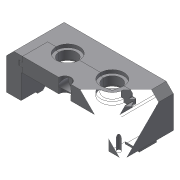
# Autodesk Inventor part: Carriage nozzel Holder
Saved by Autodesk Inventor 2015 (Build 190159000, 159)
## iProperties
Created: 2020-03-28
Part Number: Carriage nozzel Holder
Material: Generic
Document SubType Name: Modeling
Designer: Ghassan Yusuf
Density: 1 g/cm^3
Appearance: Default
Author: Ghassan Yusuf
Autodesk Inventor part; units mm, degrees
ref_plane "YZ Plane" through (0, 0, 0) normal (1, 0, 0) x (0, 1, 0)
ref_plane "XZ Plane" through (0, 0, 0) normal (0, 1, 0) x (-1, 0, 0)
ref_plane "XY Plane" through (0, 0, 0) normal (0, 0, 1) x (1, 0, 0)
sketch "Sketch1" plane through (0, 0, 0) normal (0, 0, 1) x (1, 0, 0)
  line L0 (-40.5, 17.5) -> (40.5, 17.5)
  line L1 (40.5, 17.5) -> (40.5, -17.5)
  line L2 (40.5, -17.5) -> (-40.5, -17.5)
  line L3 (-40.5, -17.5) -> (-40.5, 17.5)
  line L4 (-40.5, 17.5) -> (40.5, -17.5) construction
  line L5 (40.5, 17.5) -> (-40.5, -17.5) construction
  circle A0 centre (-15.5, 0) radius 6.125
  circle A1 centre (15.5, 0) radius 6.125
  point P0 (0, 0)
  dimension "d0" = 81
  dimension "d1" = 35
  dimension "d2" = 12.25
  dimension "d3" = 31
  dimension "d4" = 15.5
  constraints: 12 end point, 2 centre point, 2 midpoint, 2 parallel, 1 equal radius, 1 horizontal, 1 perpendicular
  measures "d0" distance of L1.end L2.end
  measures "d1" distance of L0.end L1.end
  measures "d2" diameter of A0
  measures "d3" distance of A1.centre A0.centre
  measures "d4" distance of point (0, 0) A0.centre
extrude "Extrusion1" add sketch "Sketch1" along normal mid plane 10
sketch "Sketch2" plane through (0, 0, 5) normal (0, 0, 1) x (1, 0, 0)
  circle A0 centre (-15.5, 0) radius 6.125 projected
  circle A1 centre (-15.5, 0) radius 8.125
  circle A2 centre (15.5, 0) radius 6.125 projected
  circle A3 centre (15.5, 0) radius 8.125
  point P0 (0, 0)
  dimension "d7" = 16.25
  dimension "d8" = 16.25
  constraints: 2 centre point, 2 coincident
  measures "d7" diameter of A1
  measures "d8" diameter of A3
extrude "Extrusion2" cut sketch "Sketch2" against normal blind 2.25 contours A0 | A1 | A2 | A3
sketch "Sketch3" plane through (0, 0, -5) normal (0, 0, -1) x (-1, 0, 0)
  circle A0 centre (15.5, 0) radius 8.125 projected
  circle A1 centre (15.5, 0) radius 8.125
  circle A2 centre (-15.5, 0) radius 6.125 projected
  circle A3 centre (-15.5, 0) radius 8.125
  circle A4 centre (-15.5, 0) radius 8.125 projected
  point P0 (0, 0)
  constraints: 2 centre point, 2 coincident, 2 concentric
extrude "Extrusion3" cut sketch "Sketch3" against normal blind 2.25
sketch "Sketch4" plane through (0, 0, 5) normal (0, 0, 1) x (1, 0, 0)
  line L0 (40.5, -17.5) -> (-40.5, -17.5) projected
  line L1 (-40.5, 17.5) -> (-30.5, 17.5)
  line L2 (-30.5, 17.5) -> (-30.5, -17.5)
  line L3 (-30.5, -17.5) -> (-40.5, -17.5)
  line L4 (-40.5, -17.5) -> (-40.5, 17.5)
  line L5 (40.5, 17.5) -> (30.5, 17.5)
  line L6 (30.5, 17.5) -> (30.5, -17.5)
  line L7 (30.5, -17.5) -> (40.5, -17.5)
  line L8 (40.5, -17.5) -> (40.5, 17.5)
  point P0 (0, 0)
  dimension "d13" = 10
  dimension "d14" = 10
  constraints: 16 end point, 4 parallel, 2 horizontal, 2 perpendicular, 2 point on line
  measures "d13" distance of L2.end L3.end
  measures "d14" distance of L7.end L6.end
extrude "Extrusion4" add sketch "Sketch4" along normal blind 17.17
sketch "Sketch5" plane through (0, 0, 22.17) normal (0, 0, 1) x (1, 0, 0)
  line L0 (-40.5, -17.5) -> (-40.5, 17.5) projected
  line L1 (-30.5, -17.5) -> (-30.5, 17.5) projected
  line L2 (-40.5, -6) -> (-30.5, -6)
  line L3 (-30.5, -6) -> (-30.5, 6)
  line L4 (-30.5, 6) -> (-40.5, 6)
  line L5 (-40.5, 6) -> (-40.5, -6)
  line L6 (30.5, 17.5) -> (30.5, -17.5) projected
  line L7 (30.5, -6) -> (40.3218, -6)
  line L8 (40.3218, -6) -> (40.3218, 6)
  line L9 (40.3218, 6) -> (30.5, 6)
  line L10 (30.5, 6) -> (30.5, -6)
  point P0 (0, 0)
  point P1 (-30.5, 0)
  point P2 (30.5, 0)
  dimension "d17" = 12
  constraints: 16 end point, 4 parallel, 3 point on line, 2 collinear, 2 horizontal, 2 horizontal alignment, 2 midpoint, 2 perpendicular
  measures "d17" distance between parallel lines of L4 L2
extrude "Extrusion5" add sketch "Sketch5" along normal blind 1.4
sketch "Sketch6" plane through (0, 0, -5) normal (0, 0, -1) x (-1, 0, 0)
  line L0 (-30.5, 17.5) -> (30.5, 17.5) projected
  circle A0 centre (0, 17.5) radius 4.25
  point P0 (0, 0)
  dimension "d20" = 8.5
  constraints: 1 centre point, 1 midpoint
  measures "d20" diameter of A0
extrude "Extrusion6" cut sketch "Sketch6" against normal blind 12.75
chamfer "Chamfer3" distance 5 angle 45 2 edges at (40.5, 0, -5) (-40.5, 0, -5)
fillet "Fillet4" radius 1 2 edges at (-30.5, 0, 5) (30.5, 0, 5)
sketch "Sketch7" plane through (0, 0, 5) normal (0, 0, 1) x (1, 0, 0)
  line L0 (-29.5, 17.5) -> (29.5, 17.5)
  line L1 (29.5, 17.5) -> (29.5, 0)
  line L2 (29.5, 0) -> (-29.5, 0)
  line L3 (-29.5, 0) -> (-29.5, 17.5)
  line L4 (-29.5, -17.5) -> (-29.5, 17.5) projected
  line L5 (29.5, 17.5) -> (29.5, -17.5) projected
  line L6 (-4.25, 17.5) -> (-29.5, 17.5) projected
  point P0 (0, 0)
  point P1 (0, 0)
  constraints: 8 end point, 3 collinear, 2 parallel, 1 coincident, 1 horizontal, 1 midpoint, 1 perpendicular
split body "Split1" sketch "Sketch7" result two bodies curves L2 L3 L0 L1 first body at (-4.8402, -14.3553, -4.5)
sketch "Sketch8" plane through (-7.375, 0, 5) normal (0, 1, 0) x (1, 0, 0)
  circle A0 centre (7.375, 5) radius 2
  line L0 (14.75, 10) -> (0, 10) projected
  line L1 (-2, 7.75) -> (-2, 2.25) projected
  line L2 (-19.625, 6.65) -> (-24.625, 6.65)
  line L3 (-24.625, 6.65) -> (-24.625, 3.35)
  line L4 (-24.625, 3.35) -> (-19.625, 3.35)
  line L5 (-19.625, 3.35) -> (-19.625, 6.65)
  line L6 (34.375, 6.65) -> (39.375, 6.65)
  line L7 (39.375, 6.65) -> (39.375, 3.35)
  line L8 (39.375, 3.35) -> (34.375, 3.35)
  line L9 (34.375, 3.35) -> (34.375, 6.65)
  line L10 (-14.25, 2.25) -> (-14.25, 7.75) projected
  line L11 (29, 7.75) -> (29, 2.25) projected
  line L12 (-22.125, 10) -> (-22.125, 0) projected
  line L13 (36.875, 0) -> (36.875, 10) projected
  point P0 (7.375, 10)
  point P1 (-2, 5)
  point P2 (-19.625, 5)
  point P3 (-14.25, 5)
  point P4 (34.375, 5)
  point P5 (29, 5)
  dimension "d36" = 4
  dimension "d37" = 5
  dimension "d38" = 5
  dimension "d39" = 2.5
  dimension "d40" = 2.5
  dimension "d41" = 3.3
  constraints: 16 end point, 6 midpoint, 4 parallel, 3 horizontal alignment, 2 collinear, 2 horizontal, 2 perpendicular, 1 centre point, 1 coincident, 1 vertical alignment
  measures "d36" diameter of A0
  measures "d37" distance of L2.start L2.end
  measures "d38" distance of L6.start L6.end
  measures "d39" distance between parallel lines of L5 L12
  measures "d40" distance between parallel lines of L9 L13
  measures "d41" distance of L4.end L2.start
extrude "Extrusion7" cut sketch "Sketch8" along normal blind 17.5 contours L5 L4 L12 L2 | L12 L4 L3 L2 | L6 L13 L8 L9 | L6 L7 L8 L13 bodies 2
extrude "Extrusion8" cut sketch "Sketch8" against normal blind 17.5 contours A0 bodies 2
sketch "Sketch9" plane through (-4.25, 17.5, 5) normal (0, 1, 0) x (1, 0, 0)
  line L0 (-27.4, 6.3) -> (-25.25, 6.3)
  line L1 (-25.25, 6.3) -> (-25.25, 3.7)
  line L2 (-25.25, 3.7) -> (-27.4, 3.7)
  line L3 (-27.4, 3.7) -> (-27.4, 6.3)
  line L4 (35.9, 6.3) -> (33.75, 6.3)
  line L5 (33.75, 6.3) -> (33.75, 3.7)
  line L6 (33.75, 3.7) -> (35.9, 3.7)
  line L7 (35.9, 3.7) -> (35.9, 6.3)
  line L8 (33.75, 0) -> (33.75, 10) projected
  line L9 (-25.25, 10) -> (-25.25, 0) projected
  line L10 (-25.25, 6.65) -> (-27.75, 6.65) projected
  line L11 (-27.75, 3.35) -> (-27.75, 6.65) projected
  line L12 (-25.25, 3.35) -> (-27.75, 3.35) projected
  line L13 (33.75, 6.65) -> (36.25, 6.65) projected
  line L14 (36.25, 6.65) -> (36.25, 3.35) projected
  line L15 (36.25, 3.35) -> (33.75, 3.35) projected
  point P0 (4.25, 5)
  dimension "d46" = 0.35
  dimension "d48" = 0.35
  dimension "d49" = 0.35
  dimension "d50" = 0.35
  dimension "d71" = 0.35
  constraints: 16 end point, 4 parallel, 2 collinear, 2 horizontal, 2 perpendicular, 1 point on line
  measures "d46" distance between parallel lines of L10 L0
  measures "d48" distance between parallel lines of L12 L2
  measures "d49" distance between parallel lines of L13 L4
  measures "d50" distance between parallel lines of L14 L7
  measures "d71" distance between parallel lines of L11 L3
extrude "Extrusion9" add sketch "Sketch9" against normal blind 17.5 contours L0 L1 L2 L3 | L7 L6 L5 L4 bodies 3
sketch "Sketch10" plane through (30.5, -17.5, 22.17) normal (0, -1, 0) x (1, 0, 0)
  line L0 (-32.1454, -19.32) -> (-28.8546, -19.32)
  line L1 (-28.8546, -19.32) -> (-27.2091, -22.17)
  line L2 (-27.2091, -22.17) -> (-28.8546, -25.02)
  line L3 (-28.8546, -25.02) -> (-32.1454, -25.02)
  line L4 (-32.1454, -25.02) -> (-33.7909, -22.17)
  line L5 (-33.7909, -22.17) -> (-32.1454, -19.32)
  line L6 (5, -27.17) -> (-66, -27.17) projected
  point P0 (-30.5, -22.17)
  point P1 (-30.5, -22.17)
  dimension "d54" = 5.7
  constraints: 12 end point, 1 coincident, 1 parallel, 13 other
  measures "d54" distance between parallel lines of L0 L3
extrude "Extrusion10" cut sketch "Sketch10" against normal blind 2 bodies 2
sketch "Sketch11" plane through (-7.375, 0, 5) normal (0, -1, 0) x (1, 0, 0)
  circle A0 centre (7.375, -5) radius 2
  dimension "d57" = 4
  constraints: 1 centre point, 1 coincident
  measures "d57" diameter of A0
extrude "Extrusion11" cut sketch "Sketch11" against normal blind 41.25 bodies 3
ref_plane "Work Plane1" through (-7.375, 10.5, 5) normal (0, -1, 0) x (1, 0, 0)
sketch "Sketch12" plane through (-7.375, 10.5, 5) normal (0, -1, 0) x (1, 0, 0)
  circle A0 centre (7.375, -5) radius 4.5
  dimension "d61" = 9
  constraints: 1 centre point, 1 coincident
  measures "d61" diameter of A0
extrude "Extrusion12" cut sketch "Sketch12" against normal blind 41.25 bodies 3
sketch "Sketch13" plane through (0, 0, 22.17) normal (0, 0, 1) x (1, 0, 0)
  circle A0 centre (-34, 14) radius 1.4
  circle A1 centre (-34, -14) radius 1.4
  circle A2 centre (34, 14) radius 1.4
  circle A3 centre (34, -14) radius 1.4
  line L0 (-40.5, 17.5) -> (-40.5, 6) projected
  line L1 (40.5, -17.5) -> (40.5, 17.5) projected
  point P0 (0, 0)
  dimension "d64" = 28
  dimension "d66" = 14
  dimension "d68" = 2.8
  dimension "d72" = 68
  dimension "d73" = 34
  constraints: 4 centre point, 3 equal radius, 2 horizontal alignment, 2 vertical alignment
  measures "d64" distance of A1.centre A0.centre
  measures "d66" vertical distance of point (0, 0) A0.centre
  measures "d68" diameter of A0
  measures "d72" distance of A2.centre A0.centre
  measures "d73" horizontal distance of point (0, 0) A0.centre
extrude "Extrusion13" cut sketch "Sketch13" against normal blind 13 bodies 2
equation "\"d4\" = 0.5 * d3"
equation "\"d38\" = d37"
equation "\"d39\" = 0.5 * d37"
equation "\"d40\" = 0.5 * d38"
equation "\"d48\" = d47"
equation "\"d49\" = d46"
equation "\"d50\" = d49"
equation "\"d71\" = d46"
equation "\"d66\" = 0.5 * d64"
equation "\"d73\" = 0.5 * d72"
equation "\"d47\" = d46"
body "Solid2"
body "Solid3"
